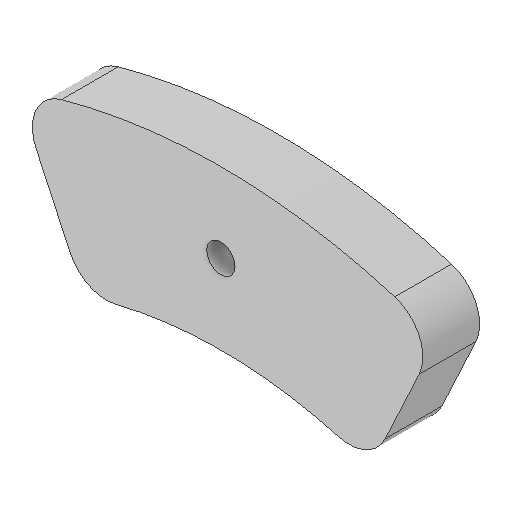
# Autodesk Inventor part: 3DP_PLA_Foot
Saved by Autodesk Inventor 2025 (Build 290162010, 162A)
## iProperties
Created: 2019-02-18
Part Number: 3DP_PLA_Foot
Material: Generic
Document SubType Name: Modeling
Designer: Andrzej
Density: 1 g/cm^3
Appearance: Default
Author: Andrzej
Autodesk Inventor part; units mm, degrees
ref_plane "YZ Plane" through (0, 0, 0) normal (1, 0, 0) x (0, 1, 0)
ref_plane "XZ Plane" through (0, 0, 0) normal (0, 1, 0) x (-1, 0, 0)
ref_plane "XY Plane" through (0, 0, 0) normal (0, 0, 1) x (1, 0, 0)
sketch "Sketch1" plane through (0, 0, 0) normal (0, 0, 1) x (1, 0, 0)
  circle A0 centre (0, 0) radius 45.5
  circle A1 centre (0, 0) radius 52.5
  circle A2 centre (0, 0) radius 38.5
  line L0 (-12.0085, 36.5793) -> (-17.9561, 49.3339)
  line L1 (13.1678, 36.1782) -> (19.101, 48.902)
  line L2 (0, 0) -> (0, 83.0319)
  point P0 (0, 45.5)
  dimension "d2" = 91
  dimension "d3" = 7
  dimension "d4" = 7
  dimension "d5" = 25
  dimension "d6" = 25
  constraints: 6 end point, 4 point on circle, 2 centre point, 1 coincident, 1 vertical, 1 vertical alignment, 2 other
  measures "d5" angle of L2 L0
  measures "d6" angle of L2 L1
extrude "Extrusion1" add sketch "Sketch1" along normal blind 5 contours L1 A2 L2 A0 | A0 L2 A1 L1 | L0 A1 L2 A0 | A0 L2 A2 L0
hole "Hole1" at (0, 45.5, 0) direction (0, 0, 1) diameter 2.5 end through all
fillet "Fillet1" radius 3.5 4 edges at (19.101, 48.902, 2.5) (13.1678, 36.1782, 2.5) (-12.0085, 36.5793, 2.5) (-17.9561, 49.3339, 2.5)
sketch "Sketch2" plane through (0, 0, 5) normal (0, 0, 1) x (1, 0, 0)
  circle A0 centre (0, 0) radius 50
  dimension "d17" = 100
  constraints: 1 centre point, 1 coincident
  measures "d17" diameter of A0
equation "\"d4\" = d3"
equation "\"d6\" = d5"
body "Solid1"
